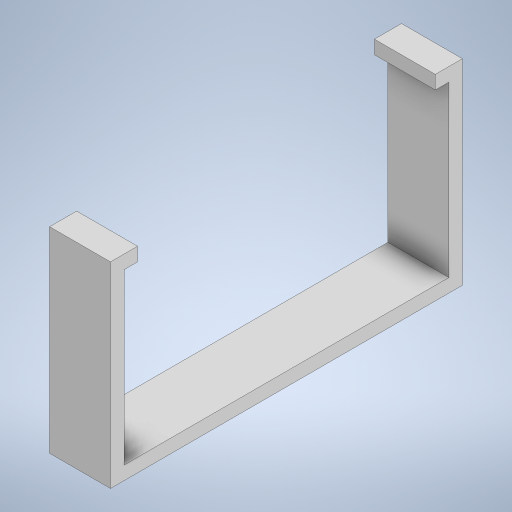
# Autodesk Inventor part: ServoHalterung_unten
Saved by Autodesk Inventor 2024 (Build 280153000, 153)
## iProperties
Created: 2023-04-25
Part Number: ServoHalterung_unten
Material: Generisch
Document SubType Name: Sheet Metal
Designer: marco
Density: 1 g/cm^3
Sheet Metal Rule: Standard_mm
Appearance: Vorgabe
Author: marco
Autodesk Inventor part; units mm, degrees
ref_plane "YZ Plane" through (0, 0, 0) normal (1, 0, 0) x (0, 1, 0)
ref_plane "XZ Plane" through (0, 0, 0) normal (0, 1, 0) x (-1, 0, 0)
ref_plane "XY Plane" through (0, 0, 0) normal (0, 0, 1) x (1, 0, 0)
sketch "Skizze1" plane through (0, 0, 0) normal (0, 1, 0) x (-1, 0, 0)
  line L0 (0, 0) -> (12, 0)
  line L1 (12, 0) -> (12, -26)
  line L2 (12, -26) -> (0, -26)
  line L3 (0, -26) -> (0, 0)
  dimension "d0" = 12
  dimension "d1" = 26
  constraints: 8 end point, 2 parallel, 1 horizontal, 1 perpendicular
  measures "d0" distance of L1.end L2.end
  measures "d1" distance of L0.end L1.end
extrude "Extrusion1" add sketch "Skizze1" along normal blind 1
sketch "Skizze2" plane through (0, 0, 0) normal (1, 0, 0) x (0, 0, -1)
  line L0 (26, 1) -> (0, 1) projected
  line L1 (0, 1) -> (0, 14.5)
  line L2 (0, 1) -> (13.5, 1) construction
  line L3 (0, 14.5) -> (2, 14.5)
  line L4 (2, 14.5) -> (2, 13.5)
  line L5 (2, 13.5) -> (1, 13.5)
  line L6 (1, 13.5) -> (1, 1)
  line L7 (0, 1) -> (1, 1)
  line L8 (24, 14.5) -> (26, 14.5)
  line L9 (26, 14.5) -> (26, 1)
  line L10 (26, 1) -> (25, 1)
  line L11 (25, 1) -> (25, 13.5)
  line L12 (25, 13.5) -> (24, 13.5)
  line L13 (24, 13.5) -> (24, 14.5)
  line L14 (25, 1) -> (26, 1)
  line L15 (26, 0) -> (26, 1) projected
  point P0 (0, 0)
  dimension "d4" = 13.5
  dimension "d5" = 90
  dimension "d6" = 2
  dimension "d7" = 1
  dimension "d8" = 1
  dimension "d9" = 2
  dimension "d10" = 24
  dimension "d11" = 1
  dimension "d12" = 13.5
  dimension "d13" = 0
  constraints: 28 end point, 11 perpendicular, 8 point on line, 1 horizontal
  measures "d4" distance of L1.start L1.end
  measures "d5" angle of L2 L1
  measures "d6" distance of L1.end L3.end
  measures "d7" distance of L3.end L4.end
  measures "d8" distance of L4.end L5.end
  measures "d9" distance of L8.start L8.end
  measures "d10" distance between parallel lines of L11 L6
  measures "d11" distance of L9.end L10.end
  measures "d12" distance of L8.end L9.end
  measures "d13" distance between parallel lines of L15 L9
extrude "Extrusion2" add sketch "Skizze2" against normal blind 12
sketch "Skizze3" plane through (-12, 0, 0) normal (0, 0, 1) x (1, 0, 0)
  line L0 (0, 0) -> (0, 14.5) projected
  line L1 (0, 0) -> (4, 0)
  line L2 (4, 0) -> (4, 1)
  line L3 (4, 1) -> (0, 1)
  line L4 (0, 1) -> (0, 0)
  line L5 (12, 14.5) -> (0, 14.5) projected
  line L6 (5, 14.5) -> (7.5, 14.5)
  line L7 (7.5, 14.5) -> (7.5, 1)
  line L8 (5, 14.5) -> (5, 1)
  line L9 (5, 1) -> (7.5, 1)
  line L10 (12, 0) -> (12, 14.5) projected
  dimension "d16" = 4
  dimension "d17" = 1
  dimension "d18" = 2.5
  dimension "d19" = 13.5
  dimension "d20" = 13.5
  dimension "d21" = 2.5
  dimension "d22" = 90
  dimension "d23" = 4.5
  constraints: 16 end point, 2 parallel, 2 perpendicular, 2 point on line, 1 horizontal, 1 vertical
  measures "d16" distance of L3.end L2.end
  measures "d17" distance of L2.end L1.end
  measures "d18" distance of L6.start L6.end
  measures "d19" distance of L6.end L7.end
  measures "d20" distance of L6.start L8.end
  measures "d21" distance of L8.end L7.end
  measures "d22" angle of L9 L8
  measures "d23" distance between parallel lines of L10 L7
extrude "Extrusion3" cut sketch "Skizze3" against normal blind 26.5
sketch "Skizze4" plane through (0, 0, 0) normal (0, 0, 1) x (1, 0, 0)
  line L0 (-4.5, 1) -> (-4.5, 14.5) projected
  line L1 (-4.5, 14.5) -> (-16.7717, 14.5)
  line L2 (-16.7717, 14.5) -> (-16.7717, 0)
  line L3 (-16.7717, 0) -> (-4.5, 0)
  line L4 (-4.5, 0) -> (-4.5, 14.5)
  point P0 (0, 0)
  constraints: 8 end point, 2 parallel, 1 horizontal, 1 perpendicular
extrude "Extrusion4" cut sketch "Skizze4" against normal blind 26.5
equation "\"Biegeradius\" = Stärke"
equation "\"BreiteBiegungsfreistellung\" = Stärke"
equation "\"TiefeBiegungsfreistellung\" = 0.5 * Stärke"
equation "\"GrößeEckenfreistellung\" = 4 * Stärke"
equation "\"MinimalRest\" = 2 * Stärke"
equation "\"Übergangsradius\" = Biegeradius"
equation "\"JacobiRadiusGröße\" = Biegeradius"
equation "\"Abstandsgröße\" = Stärke"
equation "\"Stärke\" = 0.5"
